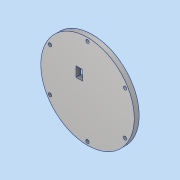
# Autodesk Inventor part: foreElectronicsSealingDisc
Saved by Autodesk Inventor 2017 (Build 210142000, 142)
## iProperties
Created: 2016-12-09
Part Number: foreElectronicsSealingDisc
Material: Aluminum 6061
Document SubType Name: Modeling
Designer: techn
Density: 2.7 g/cm^3
Appearance: Aluminum - Flat
Author: techn
Autodesk Inventor part; units mm, degrees
ref_plane "YZ Plane" through (0, 0, 0) normal (1, 0, 0) x (0, 1, 0)
ref_plane "XZ Plane" through (0, 0, 0) normal (0, 1, 0) x (-1, 0, 0)
ref_plane "XY Plane" through (0, 0, 0) normal (0, 0, 1) x (1, 0, 0)
sketch "Sketch1" plane through (0, 0, 0) normal (0, 0, 1) x (1, 0, 0)
  circle A0 centre (0, 0) radius 45.212
  dimension "d0" = 90.424
  constraints: 1 centre point, 1 coincident
  measures "d0" diameter of A0
extrude "Extrusion1" add sketch "Sketch1" along normal blind 4.7625
sketch "Sketch2" plane through (0, 0, 4.7625) normal (0, 0, 1) x (1, 0, 0)
  line L0 (0, 0) -> (0, 41.91)
  circle A0 centre (0, 41.91) radius 1.5875
  circle A1 centre (-36.2951, 20.955) radius 1.5875
  circle A2 centre (-36.2951, -20.955) radius 1.5875
  circle A3 centre (0, -41.91) radius 1.5875
  circle A4 centre (36.2951, -20.955) radius 1.5875
  circle A5 centre (36.2951, 20.955) radius 1.5875
  dimension "d3" = 41.91
  dimension "d4" = 3.175
  dimension "d7" = 360
  constraints: 6 centre point, 2 end point, 1 coincident, 1 vertical, 13 other
  measures "d3" distance of L0.start L0.end
  measures "d4" diameter of A0
extrude "Extrusion2" cut sketch "Sketch2" against normal blind 4.7625
sketch "Sketch3" plane through (0, 0, 4.7625) normal (0, 0, 1) x (1, 0, 0)
  line L0 (-11.1125, 15.875) -> (-4.7625, 15.875)
  line L1 (-4.7625, 15.875) -> (-4.7625, 6.35)
  line L2 (-4.7625, 6.35) -> (-11.1125, 6.35)
  line L3 (-11.1125, 6.35) -> (-11.1125, 15.875)
  point P0 (0, 0)
  dimension "d11" = 9.525
  dimension "d12" = 6.35
  dimension "d13" = 4.7625
  dimension "d14" = 6.35
  constraints: 8 end point, 2 parallel, 1 horizontal, 1 perpendicular
  measures "d11" distance of L2.end L0.start
  measures "d12" distance of L0.start L0.end
  measures "d13" distance from line of point (0, 0) L1
  measures "d14" distance from line of point (0, 0) L2
extrude "Extrusion3" cut sketch "Sketch3" against normal blind 4.7625
body "Solid1"
